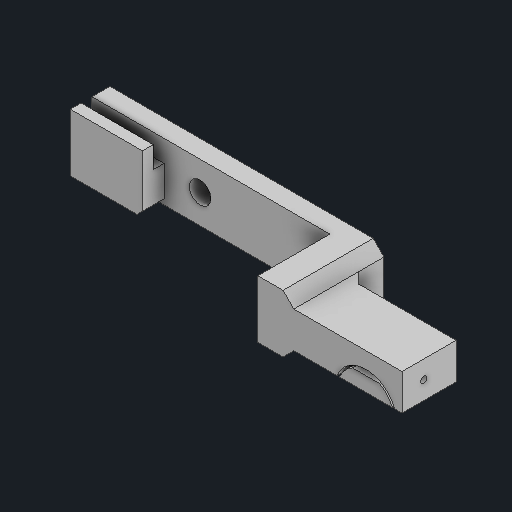
# Autodesk Inventor part: Upper probe arm
Saved by Autodesk Inventor 2026 (Build 300175050, 175E)
## iProperties
Created: 2025-07-01
Part Number: Upper probe arm
Material: Generic
Document SubType Name: Modeling
Designer: Tobymegacat
Density: 1 g/cm^3
Appearance: Default
Author: Tobymegacat
Autodesk Inventor part; units mm, degrees
ref_plane "YZ Plane" through (0, 0, 0) normal (1, 0, 0) x (0, 1, 0)
ref_plane "XZ Plane" through (0, 0, 0) normal (0, 1, 0) x (-1, 0, 0)
ref_plane "XY Plane" through (0, 0, 0) normal (0, 0, 1) x (1, 0, 0)
sketch "Sketch1" plane through (0, 0, 0) normal (0, 0, 1) x (1, 0, 0)
  line L0 (0, 0) -> (-38, 0)
  line L1 (-38, 0) -> (-38, 8)
  line L2 (-38, 8) -> (0, 8)
  line L3 (0, 8) -> (0, 0)
  dimension "d0" = 38
  dimension "d1" = 8
  constraints: 8 end point, 2 parallel, 1 horizontal, 1 perpendicular
  measures "d0" distance of L1.end L2.end
  measures "d1" distance of L0.end L1.end
extrude "Extrusion1" add sketch "Sketch1" along normal blind 2.5
sketch "Sketch2" plane through (0, 0, 2.5) normal (0, 0, 1) x (1, 0, 0)
  line L0 (0, 0) -> (-5, 0)
  line L1 (-5, 0) -> (-5, 8)
  line L2 (-5, 8) -> (0, 8)
  line L3 (0, 8) -> (0, 0)
  dimension "d4" = 5
  dimension "d5" = 8
  constraints: 8 end point, 2 parallel, 1 horizontal, 1 perpendicular
  measures "d4" distance of L1.end L2.end
  measures "d5" distance of L0.end L1.end
extrude "Extrusion2" add sketch "Sketch2" along normal blind 10
sketch "Sketch3" plane through (0, 0, 0) normal (1, 0, 0) x (0, 0, -1)
  line L0 (0, 8) -> (-12.5, 8) projected
  line L1 (-12.5, 0) -> (-12.5, 8) projected
  point P0 (0, 0)
  point P1 (-9.5, 4)
  dimension "d8" = 4
  dimension "d9" = 3
  measures "d8" distance from line of L0 point (-9.5, 4)
  measures "d9" distance from line of L1 point (-9.5, 4)
hole "Hole1" at (0, 4, 9.5) direction (-1, 0, 0) diameter 2.7 depth 10
sketch "Sketch4" plane through (0, 0, 2.5) normal (0, 0, 1) x (1, 0, 0)
  line L0 (-5, 8) -> (-38, 8) projected
  line L1 (-38, 8) -> (-38, 0) projected
  point P0 (0, 0)
  point P1 (-23, 4)
  dimension "d25" = 4
  dimension "d35" = 15
  measures "d25" distance from line of L0 point (-23, 4)
  measures "d35" distance from line of L1 point (-23, 4)
hole "Hole2" at (-23, 4, 2.5) direction (0, 0, -1) diameter 3 depth 10
sketch "Sketch5" plane through (0, 0, 2.5) normal (0, 0, 1) x (1, 0, 0)
  point P0 (0, 0)
sketch "Sketch6" plane through (0, 0, 2.5) normal (0, 0, 1) x (1, 0, 0)
  line L0 (0, 8) -> (-38, 8) projected
  line L1 (-28, 8) -> (-38, 8)
  line L2 (-38, 8) -> (-38, 0)
  line L3 (-38, 0) -> (-28, 0)
  line L4 (-28, 0) -> (-28, 8)
  point P0 (0, 0)
  point P1 (-17.4035, 8)
  dimension "d29" = 10
  constraints: 8 end point, 2 parallel, 2 point on line, 1 horizontal, 1 perpendicular
  measures "d29" distance of L2.end L3.end
extrude "Extrusion3" add sketch "Sketch6" along normal blind 3
sketch "Sketch7" plane through (-38, 8, 0) normal (0, 1, 0) x (1, 0, 0)
  line L0 (10, -2.5) -> (10, -5.5) projected
  line L1 (10, -2.5) -> (33, -2.5) projected
  line L2 (10, -2.5) -> (10, -4)
  line L3 (0, 0) -> (0, -5.5) projected
  line L4 (10, -2.5) -> (0, -2.5)
  line L5 (0, -2.5) -> (0, -4)
  line L6 (0, -4) -> (10, -4)
  line L7 (10, -4) -> (10, -2.5)
  point P0 (38, 0)
  constraints: 10 end point, 2 parallel, 1 horizontal, 1 midpoint, 1 perpendicular, 1 point on line
extrude "Extrusion4" cut sketch "Sketch7" against normal blind 3
chamfer "Chamfer1" distance 0.75 angle 45 1 edges at (-28, 0, 4)
sketch "Sketch8" plane through (0, 0, 0) normal (1, 0, 0) x (0, 0, -1)
  line L0 (-12.5, 0) -> (-12.5, 8) projected
  line L1 (-12.5, 1.5) -> (-5, 1.5)
  line L2 (-5, 1.5) -> (-5, 6.5)
  line L3 (-5, 6.5) -> (-12.5, 6.5)
  line L4 (-12.5, 6.5) -> (-12.5, 1.5)
  circle A0 centre (-9.5, 4) radius 1.35
  circle A1 centre (-9.5, 4) radius 1.35 projected
  line L5 (0, 8) -> (-12.5, 8) projected
  point P0 (0, 0)
  dimension "d36" = 5
  dimension "d37" = 7.5
  dimension "d41" = 2.7
  dimension "d48" = 1.5
  constraints: 8 end point, 2 parallel, 1 centre point, 1 concentric, 1 horizontal, 1 perpendicular, 1 point on line
  measures "d36" distance of L1.end L2.end
  measures "d37" distance of L2.end L3.end
  measures "d41" diameter of A0
  measures "d48" distance between parallel lines of L5 L3
extrude "Extrusion5" add sketch "Sketch8" along normal blind 5
sketch "Sketch9" plane through (5, 0, 0) normal (1, 0, 0) x (0, 0, -1)
  point P0 (0, 0)
sketch "Sketch10" plane through (5, 0, 0) normal (1, 0, 0) x (0, 0, -1)
  line L0 (-5, 1.5) -> (-12.5, 1.5) projected
  line L1 (-12.5, 6.5) -> (-12.5, 8) projected
  line L2 (-5, 1.5) -> (-12.5, 1.5)
  line L3 (-12.5, 1.5) -> (-12.5, 6.5)
  line L4 (-12.5, 6.5) -> (-5, 6.5)
  line L5 (-5, 6.5) -> (-5, 1.5)
  circle A0 centre (-9.5, 4) radius 0.45
  circle A1 centre (-9.5, 4) radius 1.35 projected
  point P0 (0, 0)
  point P1 (-12.5, 1.5)
  dimension "d42" = 0.9
  constraints: 8 end point, 2 parallel, 1 centre point, 1 concentric, 1 horizontal, 1 perpendicular
  measures "d42" diameter of A0
extrude "Extrusion6" add sketch "Sketch10" along normal blind 10 contours L0 L3 L4 L5 | A1
chamfer "Chamfer2" distance 1.5 angle 45 2 edges at (0, 8, 6.25) (0, 0, 6.25)
sketch "Sketch11" plane through (0, 0, 12.5) normal (0, 0, 1) x (1, 0, 0)
  line L0 (15, 1.5) -> (15, 6.5) projected
  line L1 (15, 3.5) -> (5, 3.5)
  line L2 (5, 3.5) -> (5, 4.5)
  line L3 (5, 4.5) -> (15, 4.5)
  line L4 (15, 4.5) -> (15, 3.5)
  line L5 (0, 6.5) -> (15, 6.5) projected
  arc A0 (14, 1.5) -> (6, 1.5) centre (10, 0) ccw
  line L6 (0, 1.5) -> (15, 1.5) projected
  arc A1 (13.7191, 1.3947) -> (6.2809, 1.3947) centre (10, 0) ccw
  point P0 (0, 0)
  point P1 (6, 6.5)
  point P2 (6.3221, 1.5)
  point P3 (8.122, 3.5)
  point P4 (11.878, 3.5)
  point P5 (13.6779, 1.5)
  dimension "d49" = 10
  dimension "d50" = 1
  dimension "d51" = 2
  dimension "d61" = 1
  dimension "d62" = 1
  dimension "d63" = 1.5
  dimension "d64" = 0.3
  constraints: 8 end point, 4 point on circle, 4 point on line, 2 centre point, 2 parallel, 1 horizontal, 1 perpendicular
  measures "d49" distance of L1.start L1.end
  measures "d50" distance between parallel lines of L3 L1
  measures "d51" distance between parallel lines of L5 L3
  measures "d61" distance from line of L2 A0.end
  measures "d62" distance from line of A0.start L0
  measures "d63" distance from line of L6 A0.centre
  measures "d64" radial gap between concentric circles of A0 A1
extrude "Extrusion7" cut sketch "Sketch11" against normal blind 5 contours L6 A1 L1 A0 | L1 A1 A0 | L1 A1 | L1 A1 L6 A0
chamfer "Chamfer3" distance 1.5 angle 45 1 edges at (0, 4, 5)
body "Solid1"
